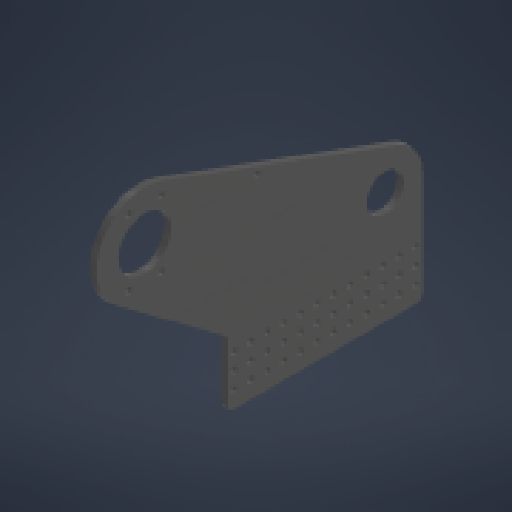
# Autodesk Inventor part: CHAPA FIXAÇÃO ESQUERDA 1 V2
Saved by Autodesk Inventor 2026 (Build 300175000, 175)
## iProperties
Created: 2026-06-18
Part Number: CHAPA FIXAÇÃO ESQUERDA 1 V2
Material: Genérico
Document SubType Name: Modeling
Designer: DELL
Density: 1 g/cm^3
Appearance: Cinza escuro
Author: DELL
Autodesk Inventor part; units mm, degrees
ref_plane "YZ Plane" through (0, 0, 0) normal (1, 0, 0) x (0, 1, 0)
ref_plane "XZ Plane" through (0, 0, 0) normal (0, 1, 0) x (-1, 0, 0)
ref_plane "XY Plane" through (0, 0, 0) normal (0, 0, 1) x (1, 0, 0)
sketch "Esboço1" plane through (0, 0, 0) normal (1, 0, 0) x (0, 1, 0)
  line L0 (0, 0) -> (50.8, 0)
  line L1 (50.8, 0) -> (50.8, -86.2)
  line L2 (50.8, -86.2) -> (0, -86.2)
  line L3 (0, -86.2) -> (0, 0)
  circle A0 centre (38.1, -5) radius 2.5
  circle A1 centre (25.4, -5) radius 2.5
  circle A2 centre (12.7, -5) radius 2.5
  circle A3 centre (38.1, -17.7) radius 2.5
  circle A4 centre (25.4, -17.7) radius 2.5
  circle A5 centre (12.7, -17.7) radius 2.5
  circle A6 centre (38.1, -30.4) radius 2.5
  circle A7 centre (25.4, -30.4) radius 2.5
  circle A8 centre (12.7, -30.4) radius 2.5
  circle A9 centre (38.1, -43.1) radius 2.5
  circle A10 centre (25.4, -43.1) radius 2.5
  circle A11 centre (12.7, -43.1) radius 2.5
  circle A12 centre (38.1, -55.8) radius 2.5
  circle A13 centre (25.4, -55.8) radius 2.5
  circle A14 centre (12.7, -55.8) radius 2.5
  circle A15 centre (38.1, -68.5) radius 2.5
  circle A16 centre (25.4, -68.5) radius 2.5
  circle A17 centre (12.7, -68.5) radius 2.5
  circle A18 centre (38.1, -81.2) radius 2.5
  circle A19 centre (25.4, -81.2) radius 2.5
  circle A20 centre (12.7, -81.2) radius 2.5
  dimension "d0" = 50.8
  dimension "d1" = 86.2
  dimension "d2" = 5
  dimension "d3" = 5
  dimension "d4" = 5
  dimension "d5" = 5
  dimension "d6" = 5
  dimension "d7" = 5
  dimension "d8" = 12.7
  dimension "d9" = 12.7
  dimension "d10" = 12.7
  dimension "d13" = 12.7
  constraints: 21 centre point, 8 end point, 2 parallel, 1 horizontal, 1 perpendicular, 1 vertical, 36 other
  measures "d0" distance of L1.end L2.end
  measures "d1" distance of L0.end L1.end
  measures "d2" diameter of A0
  measures "d3" diameter of A1
  measures "d4" diameter of A2
  measures "d5" distance from line of L0 A0.centre
  measures "d6" distance from line of L0 A1.centre
  measures "d7" distance from line of L0 A2.centre
  measures "d8" distance from line of L3 A2.centre
  measures "d9" distance of A1.centre A2.centre
  measures "d10" distance of A1.centre A0.centre
  measures "d13" distance of A0.centre A3.centre
extrude "Extrusão1" add sketch "Esboço1" along normal blind 5
sketch "Esboço2" plane through (0, 0, 0) normal (-1, 0, 0) x (0, 0, 1)
  line L0 (-86.2, 0) -> (-149.7, 0)
  line L1 (-149.7, 0) -> (-149.7, 50.8)
  line L2 (-149.7, 50.8) -> (-86.2, 50.8)
  line L3 (-86.2, 50.8) -> (-86.2, 0)
  circle A0 centre (-144.7, 38.1) radius 2.5 projected
  circle A1 centre (-144.7, 25.4) radius 2.5 projected
  circle A2 centre (-144.7, 12.7) radius 2.5 projected
  circle A3 centre (-132, 12.7) radius 2.5 projected
  circle A4 centre (-132, 25.4) radius 2.5 projected
  circle A5 centre (-132, 38.1) radius 2.5 projected
  circle A6 centre (-119.3, 38.1) radius 2.5 projected
  circle A7 centre (-119.3, 25.4) radius 2.5 projected
  circle A8 centre (-119.3, 12.7) radius 2.5 projected
  circle A9 centre (-106.6, 12.7) radius 2.5 projected
  circle A10 centre (-93.9, 12.7) radius 2.5 projected
  circle A11 centre (-93.9, 25.4) radius 2.5 projected
  circle A12 centre (-106.6, 25.4) radius 2.5 projected
  circle A13 centre (-106.6, 38.1) radius 2.5 projected
  circle A14 centre (-93.9, 38.1) radius 2.5 projected
  point P0 (0, 0)
  dimension "d20" = 50.8
  dimension "d21" = 5
  constraints: 8 end point, 2 parallel, 1 horizontal, 1 perpendicular
  measures "d20" distance of L0.end L1.end
  measures "d21" distance from line of A0.centre L1
extrude "Extrusão2" add sketch "Esboço2" against normal blind 5
sketch "Esboço3" plane through (0, 0, 0) normal (-1, 0, 0) x (0, 0, 1)
  circle A0 centre (-121.1, 85.9607) radius 4.5847 projected
  circle A1 centre (63.725, 144.496) radius 17.5 projected
  circle A2 centre (51.025, 169.896) radius 2.5 projected
  circle A3 centre (76.425, 169.896) radius 2.5 projected
  circle A4 centre (76.425, 119.096) radius 2.5 projected
  circle A5 centre (51.025, 119.096) radius 2.5 projected
  circle A6 centre (-121.1, 85.9607) radius 14.25
  circle A7 centre (63.725, 144.496) radius 20
  line L0 (-149.7, 50.8) -> (0, 50.8) projected
  line L1 (-149.7, 50.8) -> (-149.7, 85.9607)
  arc A8 (86.0063, 114.3333) -> (50.7735, 179.6885) centre (63.725, 144.496) ccw
  arc A9 (-130.9776, 112.8008) -> (-149.7, 85.9607) centre (-121.1, 85.9607) ccw
  line L2 (50.7735, 179.6885) -> (-130.9776, 112.8008)
  line L3 (0, 50.8) -> (0, 0) projected
  line L4 (0, 50.8) -> (86.0063, 114.3333)
  dimension "d26" = 28.5
  dimension "d27" = 40
  dimension "d28" = 75
  constraints: 6 end point, 4 centre point, 4 coincident, 4 point on circle, 4 tangent, 1 vertical
  measures "d26" diameter of A6
  measures "d27" diameter of A7
  measures "d28" diameter of A8
extrude "Extrusão3" add sketch "Esboço3" against normal blind 5 contours L1 A9 L2 A8 L4 L0
fillet "Arredondamento1" radius 5 3 edges at (2.5, 50.8, 0) (2.5, 0, 0) (2.5, 0, -149.7)
sketch "Esboço4" plane through (0, 0, 0) normal (-1, 0, 0) x (0, 0, 1)
  line L0 (-233.5954, 270.0952) -> (45.2176, 111.8812) projected
  line L1 (50.7735, 179.6885) -> (-130.9776, 112.8008) projected
  circle A0 centre (-22.4585, 147.4099) radius 2.5
  point P0 (0, 0)
  dimension "d34" = 5
  dimension "d35" = 5
  constraints: 1 centre point, 1 tangent
  measures "d34" diameter of A0
  measures "d35" distance from line of L1 A0.centre
extrude "Extrusão4" cut sketch "Esboço4" against normal through all
equation "\"d6\" = d5"
equation "\"d7\" = d6"
equation "\"d9\" = d8"
equation "\"d10\" = d9"
